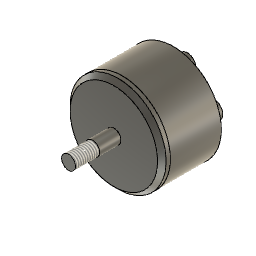
BH101_900KV_V1 v1 (Autodesk Fusion 360 design; units mm, degrees)
Autodesk Fusion 360 part; units mm, degrees
note: some values were not read from the file. Chosen so that the rebuilt part matches the saved one: which bodies a step acts on; how an offset face is resized. Set by a fixed rule: which sketch regions a step uses.
sketch "Sketch1" plane through (0, 0, 0) normal (0, 1, 0) x (1, 0, 0)
  circle A0 centre (0, 0) radius 16.95
  circle A1 centre (0, 0) radius 9.5
  circle A2 centre (-9.5, 0) radius 1.5
  circle A3 centre (0, -9.5) radius 1.5
  circle A4 centre (9.5, 0) radius 1.5
  circle A5 centre (0, 9.5) radius 1.5
  circle A6 centre (0, 0) radius 2.5
  circle A7 centre (0, 0) radius 7
  circle A8 centre (0, 0) radius 12.5
  circle A9 centre (0, -9.5) radius 3
  circle A10 centre (-9.5, 0) radius 3
  circle A11 centre (9.5, 0) radius 3
  circle A12 centre (0, 9.5) radius 3
  line L0 (-3, -9.5) -> (-3, -6.3246)
  line L1 (3, -9.5) -> (3, -6.3246)
  line L2 (9.5, -3) -> (6.3246, -3)
  line L3 (9.5, 3) -> (6.3246, 3)
  line L4 (-9.5, -3) -> (-6.3246, -3)
  line L5 (-9.5, 3) -> (-6.3246, 3)
  line L6 (3, 9.5) -> (3, 6.3246)
  line L7 (-3, 9.5) -> (-3, 6.3246)
  point P0 (0, -9.5)
  point P1 (0, 9.5)
  point P2 (9.5, 0)
  point P3 (-9.5, 0)
  dimension "d1" = 33.9
  dimension "d2" = 19
  dimension "d3" = 3
  dimension "d4" = 3
  dimension "d5" = 3
  dimension "d6" = 3
  dimension "d7" = 5
  dimension "d25" = 25
  dimension "d26" = 14
  constraint coincident A0.centre A1.centre
  constraint coincident A1 P0
  constraint coincident A1 P1
  constraint vertical P0 P1
  constraint coincident A1 P2
  constraint coincident A1 P3
  constraint horizontal P2 P3
  constraint coincident P3 A2.centre
  constraint coincident P0 A3.centre
  constraint coincident P2 A4.centre
  constraint coincident P1 A5.centre
  constraint concentric A0 A6
  constraint concentric A6 A7
  constraint concentric A6 A8
  constraint tangent A8 A9
  constraint tangent A8 A10
  constraint tangent A8 A11
  constraint tangent A8 A12
  constraint coincident A9 L0.start
  constraint coincident A7 L0.end
  constraint tangent A9 L0
  constraint vertical L0
  constraint coincident A9 L1.start
  constraint coincident A7 L1.end
  constraint tangent A9 L1
  constraint vertical L1
  constraint coincident A11 L2.start
  constraint coincident A7 L2.end
  constraint tangent A11 L2
  constraint horizontal L2
  constraint coincident A11 L3.start
  constraint coincident A7 L3.end
  constraint tangent A11 L3
  constraint horizontal L3
  constraint coincident A10 L4.start
  constraint coincident A7 L4.end
  constraint tangent A10 L4
  constraint horizontal L4
  constraint coincident A10 L5.start
  constraint coincident A7 L5.end
  constraint tangent A10 L5
  constraint horizontal L5
  constraint coincident A12 L6.start
  constraint coincident A7 L6.end
  constraint tangent A12 L6
  constraint vertical L6
  constraint coincident A12 L7.start
  constraint coincident A7 L7.end
  constraint tangent A12 L7
  constraint vertical L7
  measures "d1" diameter of A0
  measures "d2" diameter of A1
  measures "d3" diameter of A2
  measures "d4" diameter of A3
  measures "d5" diameter of A4
  measures "d6" diameter of A5
  measures "d7" diameter of A6
  measures "d25" diameter of A8
  measures "d26" diameter of A7
extrude "Extrude1" add sketch "Sketch1" against normal blind 42 contours A6 makes body 1
extrude "Extrude2" add sketch "Sketch1" against normal blind 26 contours A0 | A1 A4 | A1 A4 | A1 A4 A7 A11 | A1 A4 A11 | A1 A7 A11 L3 | A1 A11 L3 | A1 A11 L2 | A1 A7 A11 L2 | A1 A7 L3 L6 | A1 A8 A11 A12 L3 L6 | A7 A9 A10 A11 A12 | A7 A11 | A1 A8 A9 A11 L1 L2 | A1 A7 L1 L2 | A1 A7 A12 L6 | A1 A12 L6 | A1 A9 L1 | A1 A7 A9 L1 | A1 A5 A7 A12 | A1 A5 A12 | A1 A8 A10 A12 L5 L7 | A1 A8 A9 A10 L0 L4 | A1 A3 A9 | A1 A3 A7 A9 | A1 A5 | A1 A5 | A7 A12 | A1 A2 A10 | A1 A12 L7 | A1 A9 L0 | A1 A3 | A1 A3 | A7 A9 | A1 A7 A12 L7 | A1 A10 L5 | A1 A10 L4 | A1 A7 L5 L7 | A1 A7 A9 L0 | A1 A7 L0 L4 | A1 A2 A7 A10 | A1 A7 A10 L5 | A1 A7 A10 L4 | A1 A2 | A1 A2 | A7 A10 bodies 1
extrude "Extrude3" cut sketch "Sketch1" against normal blind 4 contours A1 A4 | A1 A4 | A1 A5 | A1 A5 | A1 A3 | A1 A3 | A1 A2 | A1 A2 bodies 1
ref_plane "WorkPlane1" through (0, -5, 0) normal (0, 1, 0) x (1, 0, 0)
split "Split1" by plane through (0, -5, 0) normal (0, 1, 0) bodies 1 makes body 2 at (0.0374, 0, -2.6681)
chamfer "Chamfer1" distance 5 angle 45 1 edges at (-15.8029, -5, 6.1294) on bodies 2
ref_plane "WorkPlane2" through (0, -23, 0) normal (0, -1, 0) x (-1, 0, 0)
split "Split2" by plane through (0, -23, 0) normal (0, -1, 0) bodies 1 makes body 3 at (12.0702, -26, 0.8421)
chamfer "Chamfer2" distance 1.5 angle 45 1 edges at (-15.8029, -26, -6.1294) on bodies 3
ref_plane "WorkPlane3" through (0, -33.5, 0) normal (0, -1, 0) x (-1, 0, 0)
split "Split3" by plane through (0, -33.5, 0) normal (0, -1, 0) bodies 3 makes body 4 at (2.4876, -36.3333, 0.2489)
thread "Thread1" "ISO Metric profile 5.0 M5x0.8 6g" major diameter 4.901 minor diameter 3.9895 pitch 0.8 angle 60 resizes the face on face at (2.4876, -36.3333, 0.2489) on bodies 4
sketch "Sketch2" plane through (0, 0, 0) normal (0, 1, 0) x (1, 0, 0)
  circle A0 centre (0, 0) radius 16.95
extrude "Extrude4" add 1 faces at (0.0374, 0, -2.6681) along direction (0, -1, 0) blind 5 on bodies 2 bodies 2 3 4 1
ref_plane "WorkPlane4" through (0, -2, 0) normal (0, 1, 0) x (1, 0, 0)
split "Split4" by plane through (0, -2, 0) normal (0, 1, 0) and through (0, -5, 0) normal (0, 1, 0) bodies 2 makes body 5 at (0.0374, 0, -2.6681) makes body 6 at (16.8658, -3, 1.6877)
move_face "OffsetFaces1" offset -10 1 faces at (16.8658, -3, 1.6877) on bodies 6
extrude "Extrude5" cut sketch "Sketch1" against normal blind 2 contours A0 | A1 A7 L3 L6 | A1 A8 A11 A12 L3 L6 | A1 A8 A9 A11 L1 L2 | A1 A7 L1 L2 | A1 A8 A10 A12 L5 L7 | A1 A8 A9 A10 L0 L4 | A1 A7 L5 L7 | A1 A7 L0 L4 bodies 5
equation "d4 = d3"
equation "d5 = d3"
equation "d6 = d3"
equation "d25 = d2 + 6 mm"
equation "d26 = d2 - 5 mm"
